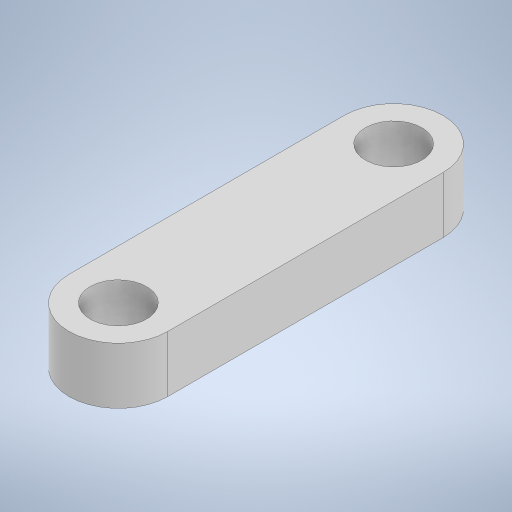
# Autodesk Inventor part: Hebel
Saved by Autodesk Inventor 2023.2 (Build 272271030, 271C)
## iProperties
Created: 2023-02-11
Part Number: Hebel
Material: Generic
Document SubType Name: Modeling
Designer: Ayush
Density: 1 g/cm^3
Appearance: Default
Author: Ayush
Autodesk Inventor part; units mm, degrees
ref_plane "YZ Plane" through (0, 0, 0) normal (1, 0, 0) x (0, 1, 0)
ref_plane "XZ Plane" through (0, 0, 0) normal (0, 1, 0) x (-1, 0, 0)
ref_plane "XY Plane" through (0, 0, 0) normal (0, 0, 1) x (1, 0, 0)
sketch "Sketch1" plane through (0, 0, 0) normal (0, 1, 0) x (-1, 0, 0)
  line L0 (7, 0) -> (7, -19.5)
  line L1 (7, 0) -> (7, 19.5)
  line L2 (-7, 0) -> (-7, -19.5)
  line L3 (-7, 0) -> (-7, 19.5)
  circle A0 centre (0, -19.5) radius 4
  circle A1 centre (0, 19.5) radius 4
  arc A2 (-7, -19.5) -> (7, -19.5) centre (0, -19.5) ccw
  arc A3 (7, 19.5) -> (-7, 19.5) centre (0, 19.5) ccw
  point P0 (0, 0)
  point P1 (0, 26.5)
  point P2 (0, -26.5)
  dimension "d0" = 7
  dimension "d1" = 7
  dimension "d2" = 19.5
  dimension "d3" = 19.5
  dimension "d6" = 14
  dimension "d7" = 14
  dimension "d8" = 8
  dimension "d9" = 8
  dimension "d10" = 14
  dimension "d13" = 14
  dimension "d14" = 39
  dimension "d15" = 53
  constraints: 8 end point, 6 point on circle, 4 centre point, 4 vertical, 1 coincident, 1 concentric
  measures "d0" distance of point (0, 0) L0.start
  measures "d1" distance of point (0, 0) L2.start
  measures "d2" distance of L0.start L0.end
  measures "d3" distance of L0.start L1.end
  measures "d6" distance of L2.end L0.end
  measures "d7" distance of L3.end L1.end
  measures "d8" diameter of A0
  measures "d9" diameter of A1
  measures "d10" diameter of A2
  measures "d13" diameter of A3
  measures "d14" distance of A1.centre A0.centre
  measures "d15" distance of point (0, 26.5) point (0, -26.5)
extrude "Extrusion1" add sketch "Sketch1" along normal blind 8
body "Solid1"
